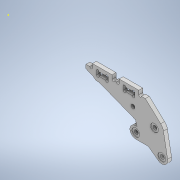
# Autodesk Inventor part: 後ろウィング固定フレーム
Saved by Autodesk Inventor 2020.2 (Build 242310000, 310)
## iProperties
Created: 2020-05-05
Part Number: 後ろウィング固定フレーム
Material: 一般
Document SubType Name: Modeling
Designer: mozar
Density: 1 g/cm^3
Appearance: 既定
Author: mozar
Autodesk Inventor part; units mm, degrees
ref_plane "YZ Plane" through (0, 0, 0) normal (1, 0, 0) x (0, 1, 0)
ref_plane "XZ Plane" through (0, 0, 0) normal (0, 1, 0) x (-1, 0, 0)
ref_plane "XY Plane" through (0, 0, 0) normal (0, 0, 1) x (1, 0, 0)
sketch "スケッチ2" plane through (0, 0, 0) normal (0, 0, 1) x (1, 0, 0)
  line L0 (-101.5, 47.999998) -> (108.5, 47.999998)
  circle A0 centre (111.885049, -19.000002) radius 4
  circle A1 centre (171.880735, -19.719469) radius 4
  circle A2 centre (111.885049, -19.000002) radius 7
  circle A3 centre (171.880735, -19.719469) radius 7
  line L1 (171.880735, -19.719469) -> (111.885049, -19.000002) construction
  line L2 (171.964673, -12.719973) -> (111.968987, -12.000505)
  line L3 (111.801111, -25.999499) -> (171.796797, -26.718966)
  arc A4 (171.796797, -26.718966) -> (171.964673, -12.719973) centre (171.880735, -19.719469) ccw
  arc A5 (111.968987, -12.000505) -> (111.801111, -25.999499) centre (111.885049, -19.000002) ccw
  line L4 (173.79611, -12.986614) -> (250.19065, -34.719469)
  circle A6 centre (241.981901, -63.574563) radius 30
  line L5 (268.180017, -78.191633) -> (221.951227, -41.241357)
  line L6 (221.951227, -41.241357) -> (169.96536, -26.452325)
  line L7 (271.981901, -113.136134) -> (271.981901, -54.819928)
  line L8 (111.885049, -19.000002) -> (111.885049, 40.999998) construction
  line L9 (118.885049, -19.000002) -> (118.885049, 40.999998)
  line L10 (104.885049, 40.999998) -> (104.885049, -19.000002)
  arc A7 (104.885049, -19.000002) -> (118.885049, -19.000002) centre (111.885049, -19.000002) ccw
  arc A8 (118.885049, 40.999998) -> (104.885049, 40.999998) centre (111.885049, 40.999998) ccw
  circle A9 centre (29.431847, 47.237971) radius 30
  line L11 (113.319325, 34.148513) -> (35.578743, 17.874462)
  line L12 (-0.558473, 47.999998) -> (57.548936, 36.777123)
  line L13 (57.548936, 36.777123) -> (110.450773, 47.851484)
  circle A10 centre (113.5, -20.000002) radius 68
  line L14 (321.963533, -82.955067) -> (60.270532, 100.284345)
  line L15 (259.189194, -39.000002) -> (111.885049, -19.000002)
  arc A11 (93.592427, -27.104845) -> (135.370976, -5.924402) centre (95.060351, 21.794105) ccw
  arc A12 (135.370976, -5.924402) -> (135.847591, -3.671647) centre (132.898992, -4.224609) ccw
  arc A13 (135.847591, -3.671647) -> (83.183341, 18.55647) centre (102.157897, -9.989602) ccw
  line L16 (111.885049, -19.000002) -> (112.689188, 40.994609) construction
  line L17 (118.88442, -19.093818) -> (119.688559, 40.900793)
  line L18 (105.689816, 41.088425) -> (104.885678, -18.906186)
  arc A14 (104.885678, -18.906186) -> (118.88442, -19.093818) centre (111.885049, -19.000002) ccw
  arc A15 (119.688559, 40.900793) -> (105.689816, 41.088425) centre (112.689188, 40.994609) ccw
  line L19 (164.994898, 47.999998) -> (164.994898, 25.999998)
  line L20 (164.994898, 25.999998) -> (327.494898, -102.000002)
  circle A16 centre (116.292557, -40.000002) radius 68
  circle A17 centre (-98.885049, -0.000002) radius 67.5
  line L21 (321.363327, -8.500986) -> (-152.668056, 78.49822)
  line L22 (104.889695, -3) -> (104.889695, 0)
  line L23 (104.889695, -3) -> (72.06562, -3)
  line L24 (72.06562, 0) -> (104.889695, 0)
  circle A18 centre (83.376901, -17.5) radius 13.85
  point P0 (0, 0)
  point P1 (141.882892, -19.359736)
  point P2 (111.885049, 10.999998)
  point P3 (105.885049, -0.000002)
  point P4 (105.885049, -0.000002)
  point P5 (23.732778, -42.728965)
  point P6 (112.287118, 10.997304)
  dimension "d31" = 8
  dimension "d32" = 8
  dimension "d33" = 3
  dimension "d34" = 3
  dimension "d35" = 60
  dimension "d36" = 14
  dimension "d37" = 14
  dimension "d38" = 60
  dimension "d39" = 14
  dimension "d40" = 60
  dimension "d41" = 14
  dimension "d42" = 6
  dimension "d43" = 35
  dimension "d44" = 13.271
  dimension "d45" = 14
  dimension "d46" = 20
  dimension "d47" = 15
  dimension "d48" = 22
  dimension "d49" = 150
  dimension "d50" = 162.5
  dimension "d51" = 0
  dimension "d52" = 136
  dimension "d53" = 136
  dimension "d54" = 135
  dimension "d55" = 38.2272
  dimension "d56" = 18
  constraints: 56 end point, 28 point on circle, 25 tangent, 18 centre point, 4 equal length, 3 coincident, 3 midpoint, 3 parallel, 3 vertical, 2 point on line, 1 concentric, 1 horizontal, 14 other
  measures "d31" diameter of A0
  measures "d32" diameter of A1
  measures "d33" radial gap between concentric circles of A0 A2
  measures "d35" distance of L1.start L1.end
  measures "d36" diameter of A5
  measures "d37" distance from line of L4 L5.end
  measures "d38" diameter of A6
  measures "d39" diameter of A8
  measures "d40" diameter of A9
  measures "d41" distance from line of L11 L12.end
  measures "d42" horizontal distance of L1.end point (105.885, 0)
  measures "d43" angle of L14 L0
  measures "d45" diameter of A15
  measures "d46" vertical distance of L15.start L1.end
  measures "d47" vertical distance of L1.start L4.end
  measures "d48" distance of L19.start L19.end
  measures "d49" vertical distance of L19.start L20.end
  measures "d50" distance from line of L19 L20.end
  measures "d51" distance from line of L19.start L0
  measures "d52" diameter of A10
  measures "d53" diameter of A16
  measures "d54" diameter of A17
  measures "d55" angle of L0 L20
  measures "d56" distance from line of L5.start L20
sketch "スケッチ1" plane through (0, 0, 0) normal (0, 0, 1) x (1, 0, 0)
  line L0 (-101.5, 47.999998) -> (108.5, 47.999998)
  circle A0 centre (111.885049, -19.000002) radius 4
  circle A1 centre (171.880735, -19.719469) radius 4
  circle A2 centre (111.885049, -19.000002) radius 7
  circle A3 centre (171.880735, -19.719469) radius 7
  line L1 (171.880735, -19.719469) -> (111.885049, -19.000002) construction
  line L2 (171.964673, -12.719973) -> (111.968987, -12.000505)
  line L3 (111.801111, -25.999499) -> (171.796797, -26.718966)
  arc A4 (171.796797, -26.718966) -> (171.964673, -12.719973) centre (171.880735, -19.719469) ccw
  arc A5 (111.968987, -12.000505) -> (111.801111, -25.999499) centre (111.885049, -19.000002) ccw
  line L4 (173.79611, -12.986614) -> (250.19065, -34.719469)
  circle A6 centre (241.981901, -63.574563) radius 30
  line L5 (268.180017, -78.191633) -> (221.951227, -41.241357)
  line L6 (221.951227, -41.241357) -> (169.96536, -26.452325)
  line L7 (271.981901, -113.136134) -> (271.981901, -54.819928)
  line L8 (111.885049, -19.000002) -> (111.885049, 40.999998) construction
  line L9 (118.885049, -19.000002) -> (118.885049, 40.999998)
  line L10 (104.885049, 40.999998) -> (104.885049, -19.000002)
  arc A7 (104.885049, -19.000002) -> (118.885049, -19.000002) centre (111.885049, -19.000002) ccw
  arc A8 (118.885049, 40.999998) -> (104.885049, 40.999998) centre (111.885049, 40.999998) ccw
  circle A9 centre (29.431847, 47.237971) radius 30
  line L11 (113.319325, 34.148513) -> (35.578743, 17.874462)
  line L12 (-0.558473, 47.999998) -> (57.548936, 36.777123)
  line L13 (57.548936, 36.777123) -> (110.450773, 47.851484)
  circle A10 centre (113.5, -20.000002) radius 68
  line L14 (321.963533, -82.955067) -> (60.270532, 100.284345)
  line L15 (259.189194, -39.000002) -> (111.885049, -19.000002)
  arc A11 (93.592427, -27.104845) -> (135.370976, -5.924402) centre (95.060351, 21.794105) ccw
  arc A12 (135.370976, -5.924402) -> (135.847591, -3.671647) centre (132.898992, -4.224609) ccw
  arc A13 (135.847591, -3.671647) -> (83.183341, 18.55647) centre (102.157897, -9.989602) ccw
  line L16 (111.885049, -19.000002) -> (112.689188, 40.994609) construction
  line L17 (118.88442, -19.093818) -> (119.688559, 40.900793)
  line L18 (105.689816, 41.088425) -> (104.885678, -18.906186)
  arc A14 (104.885678, -18.906186) -> (118.88442, -19.093818) centre (111.885049, -19.000002) ccw
  arc A15 (119.688559, 40.900793) -> (105.689816, 41.088425) centre (112.689188, 40.994609) ccw
  line L19 (164.994898, 47.999998) -> (164.994898, 25.999998)
  line L20 (164.994898, 25.999998) -> (327.494898, -102.000002)
  circle A16 centre (116.292557, -40.000002) radius 68
  circle A17 centre (-98.885049, -0.000002) radius 67.5
  line L21 (321.363327, -8.500986) -> (-152.668056, 78.49822)
  line L22 (104.889695, -3) -> (104.889695, 0)
  line L23 (72.06562, 0) -> (104.889695, 0)
  circle A18 centre (83.376901, -17.5) radius 13.85
  line L24 (104.889695, -3) -> (116.636882, -13.859955)
  line L25 (109.334849, -25.518934) -> (59.439695, -6)
  line L26 (94.885049, -3) -> (89.885049, -3)
  line L27 (87.885049, -3) -> (87.885049, -6)
  line L28 (89.885049, -6) -> (94.885049, -6)
  line L29 (96.885049, -6) -> (96.885049, -3)
  line L30 (74.439695, -3) -> (69.439695, -3)
  line L31 (67.439695, -3) -> (67.439695, -6)
  line L32 (69.439695, -6) -> (74.439695, -6)
  line L33 (76.439695, -6) -> (76.439695, -3)
  line L34 (59.439695, -3) -> (59.439695, -6)
  arc A19 (67.439695, -6) -> (69.439695, -6) centre (68.439695, -6) ccw
  arc A20 (74.439695, -6) -> (76.439695, -6) centre (75.439695, -6) ccw
  arc A21 (76.439695, -3) -> (74.439695, -3) centre (75.439695, -3) ccw
  arc A22 (69.439695, -3) -> (67.439695, -3) centre (68.439695, -3) ccw
  arc A23 (87.885049, -6) -> (89.885049, -6) centre (88.885049, -6) ccw
  arc A24 (94.885049, -6) -> (96.885049, -6) centre (95.885049, -6) ccw
  arc A25 (96.885049, -3) -> (94.885049, -3) centre (95.885049, -3) ccw
  arc A26 (89.885049, -3) -> (87.885049, -3) centre (88.885049, -3) ccw
  line L35 (104.889695, -3) -> (96.885049, -3)
  line L36 (94.885049, -3) -> (89.885049, -3)
  line L37 (87.885049, -3) -> (76.439695, -3)
  line L38 (74.439695, -3) -> (69.439695, -3)
  line L39 (67.439695, -3) -> (59.439695, -3)
  line L40 (84.885049, -3) -> (84.885049, -6)
  arc A27 (84.885049, -6) -> (91.5308, -9) centre (88.885049, -6) ccw
  line L41 (91.5308, -9) -> (93.239298, -9)
  arc A28 (93.239298, -9) -> (99.885049, -6) centre (95.885049, -6) ccw
  line L42 (99.885049, -6) -> (99.885049, -3)
  line L43 (79.439695, -3) -> (79.439695, -6)
  arc A29 (72.793944, -9) -> (79.439695, -6) centre (75.439695, -6) ccw
  line L44 (72.793944, -9) -> (71.085447, -9)
  arc A30 (64.439695, -6) -> (71.085447, -9) centre (68.439695, -6) ccw
  line L45 (64.439695, -6) -> (64.439695, -3)
  line L46 (84.885049, -3) -> (84.885049, 0)
  line L47 (84.885049, 0) -> (99.885049, 0)
  line L48 (99.885049, 0) -> (99.885049, -3)
  line L49 (87.885049, -3) -> (84.885049, -3)
  line L50 (99.885049, -3) -> (96.885049, -3)
  line L51 (94.885049, -3) -> (89.885049, -3)
  line L52 (64.439695, -3) -> (64.439695, 0)
  line L53 (64.439695, 0) -> (79.439695, 0)
  line L54 (79.439695, 0) -> (79.439695, -3)
  line L55 (79.439695, -3) -> (76.439695, -3)
  line L56 (74.439695, -3) -> (69.439695, -3)
  line L57 (67.439695, -3) -> (64.439695, -3)
  circle A31 centre (63.439695, -3) radius 1
  circle A32 centre (83.885049, -3) radius 1
  circle A33 centre (80.439695, -3) radius 1
  circle A34 centre (100.885049, -3) radius 1
  point P0 (0, 0)
  point P1 (141.882892, -19.359736)
  point P2 (111.885049, 10.999998)
  point P3 (105.885049, -0.000002)
  point P4 (105.885049, -0.000002)
  point P5 (23.732778, -42.728965)
  point P6 (112.287118, 10.997304)
  point P7 (104.889695, -1.5)
  point P8 (101.885049, -3)
  point P9 (82.885049, -3)
  point P10 (81.439695, -3)
  point P11 (62.439695, -3)
  point P12 (65.111495, -8.218802)
  point P13 (69.378847, -9.888186)
  point P14 (108.577071, -25.222492)
  point P15 (108.642416, -25.203657)
  dimension "d0" = 8
  dimension "d1" = 8
  dimension "d2" = 3
  dimension "d3" = 3
  dimension "d4" = 60
  dimension "d5" = 14
  dimension "d6" = 14
  dimension "d7" = 60
  dimension "d8" = 14
  dimension "d9" = 60
  dimension "d10" = 14
  dimension "d11" = 6
  dimension "d12" = 35
  dimension "d13" = 13.271
  dimension "d14" = 14
  dimension "d15" = 20
  dimension "d16" = 15
  dimension "d17" = 22
  dimension "d18" = 150
  dimension "d19" = 162.5
  dimension "d20" = 0
  dimension "d21" = 136
  dimension "d22" = 136
  dimension "d23" = 135
  dimension "d24" = 38.2272
  dimension "d25" = 18
  dimension "d26" = 9
  dimension "d27" = 3
  dimension "d28" = 9
  dimension "d29" = 3
  dimension "d30" = 8
  dimension "d57" = 45.45
  dimension "d58" = 3
  dimension "d60" = 2
  dimension "d61" = 2
  dimension "d62" = 2
  dimension "d63" = 2
  dimension "d64" = 2
  dimension "d65" = 2
  dimension "d66" = 2
  dimension "d67" = 2
  dimension "d68" = 3
  dimension "d69" = 3
  dimension "d73" = 8
  dimension "d74" = 2
  dimension "d75" = 2
  dimension "d76" = 2
  dimension "d77" = 2
  constraints: 122 end point, 53 point on circle, 37 tangent, 33 centre point, 17 parallel, 17 point on line, 15 horizontal, 8 perpendicular, 5 midpoint, 5 vertical, 4 equal length, 3 coincident, 30 other
  measures "d0" diameter of A0
  measures "d1" diameter of A1
  measures "d4" distance of L1.start L1.end
  measures "d5" diameter of A5
  measures "d6" distance from line of L4 L5.end
  measures "d7" diameter of A6
  measures "d8" diameter of A8
  measures "d9" diameter of A9
  measures "d10" distance from line of L11 L12.end
  measures "d11" horizontal distance of L1.end point (105.885, 0)
  measures "d12" angle of L14 L0
  measures "d14" diameter of A15
  measures "d15" vertical distance of L15.start L1.end
  measures "d16" vertical distance of L1.start L4.end
  measures "d17" distance of L19.start L19.end
  measures "d18" vertical distance of L19.start L20.end
  measures "d19" distance from line of L19 L20.end
  measures "d20" distance from line of L19.start L0
  measures "d21" diameter of A10
  measures "d22" diameter of A16
  measures "d23" diameter of A17
  measures "d24" angle of L0 L20
  measures "d25" distance from line of L5.start L20
  measures "d26" distance of L29.start L27.end
  measures "d27" distance of L27.end L27.start
  measures "d28" distance of L33.start L31.end
  measures "d29" distance of L31.end L31.start
  measures "d30" distance between parallel lines of L29 L10
  measures "d57" distance from line of L34.start L22
  measures "d58" distance of L34.start L25.end
  measures "d60" diameter of A19
  measures "d61" diameter of A20
  measures "d62" diameter of A21
  measures "d63" diameter of A22
  measures "d64" diameter of A23
  measures "d65" diameter of A24
  measures "d66" diameter of A25
  measures "d67" diameter of A26
  measures "d68" distance between parallel lines of L27 L40
  measures "d69" distance between parallel lines of L33 L43
  measures "d73" distance between parallel lines of L34 L31
  measures "d74" diameter of A31
  measures "d75" diameter of A32
  measures "d76" diameter of A33
  measures "d77" diameter of A34
extrude "押し出し1" add sketch "スケッチ1" against normal blind 3 contours A2 A11 | L35 L24 L18 L10 | L10 A2 A11 L25 A18 A28 L42 A34 L35 | L48 L35 A25 L26 A26 L37 L46 L23 | L24 L2 A2 L18 | A11 A2 | L42 A28 A18 L28 A24 L29 L35 | L24 A2 L2 | L54 L37 A21 L30 A22 L39 L52 L53 L23 | L37 L27 A18 L40 | L40 A18 A32 | L25 A18 L44 A29 L43 A33 A32 L40 A27 L41 A28 | L43 A18 L33 L37 | A33 A18 L43 | A32 A18 A33 L37 | A18 L27 A23 L28 A28 L41 A27 L40 | L25 A30 L44 A18 | L43 A29 L44 A18 A20 L33 | L44 A30 L25 L45 L39 L31 A19 L32 A20 A18 | A30 L25 | L45 A30 L25 L34 L39 A31 | A0
hole "穴1" at (111.885049, -19.000002, 0) direction (0, 0, -1) diameter 3 depth 12 tip angle 118
sketch "スケッチ3" plane through (0, 0, 0) normal (0, 0, 1) x (1, 0, 0)
  circle A0 centre (111.885049, -19.000002) radius 1.5
  line L0 (89.885049, -6) -> (94.885049, -6)
  arc A1 (94.885049, -6) -> (96.885049, -6) centre (95.885049, -6) ccw
  line L1 (96.885049, -6) -> (96.885049, -3)
  arc A2 (96.885049, -3) -> (94.885049, -3) centre (95.885049, -3) ccw
  line L2 (94.885049, -3) -> (89.885049, -3)
  arc A3 (89.885049, -3) -> (87.885049, -3) centre (88.885049, -3) ccw
  line L3 (87.885049, -3) -> (87.885049, -6)
  arc A4 (87.885049, -6) -> (89.885049, -6) centre (88.885049, -6) ccw
  arc A5 (76.439695, -3) -> (74.439695, -3) centre (75.439695, -3) ccw
  line L4 (74.439695, -3) -> (69.439695, -3)
  arc A6 (69.439695, -3) -> (67.439695, -3) centre (68.439695, -3) ccw
  line L5 (67.439695, -3) -> (67.439695, -6)
  arc A7 (67.439695, -6) -> (69.439695, -6) centre (68.439695, -6) ccw
  line L6 (69.439695, -6) -> (74.439695, -6)
  arc A8 (74.439695, -6) -> (76.439695, -6) centre (75.439695, -6) ccw
  line L7 (76.439695, -6) -> (76.439695, -3)
  line L8 (64.439695, -3) -> (64.439695, 0)
  line L9 (64.439695, 0) -> (79.439695, 0)
  line L10 (79.439695, 0) -> (79.439695, -3)
  arc A9 (79.439695, -3) -> (81.439695, -3) centre (80.439695, -3) ccw
  line L11 (81.439695, -3) -> (82.885049, -3)
  arc A10 (82.885049, -3) -> (84.885049, -3) centre (83.885049, -3) ccw
  line L12 (84.885049, -3) -> (84.885049, 0)
  line L13 (84.885049, 0) -> (99.885049, 0)
  line L14 (99.885049, 0) -> (99.885049, -3)
  arc A11 (99.885049, -3) -> (101.885049, -3) centre (100.885049, -3) ccw
  line L15 (101.885049, -3) -> (104.889695, -3)
  line L16 (104.889695, -3) -> (116.636882, -13.859955)
  arc A12 (108.642416, -25.203657) -> (116.636882, -13.859955) centre (111.885049, -19.000002) ccw
  arc A13 (108.577071, -25.222492) -> (108.642416, -25.203657) centre (95.060351, 21.794105) ccw
  line L17 (108.577071, -25.222492) -> (69.378847, -9.888186)
  arc A14 (65.111495, -8.218802) -> (69.378847, -9.888186) centre (68.439695, -6) ccw
  line L18 (65.111495, -8.218802) -> (59.439695, -6)
  line L19 (59.439695, -6) -> (59.439695, -3)
  line L20 (59.439695, -3) -> (62.439695, -3)
  arc A15 (62.439695, -3) -> (64.439695, -3) centre (63.439695, -3) ccw
  circle A16 centre (111.885049, -19.000002) radius 9
  circle A17 centre (111.885049, -19.000002) radius 9.5
  line L21 (111.801111, -25.999499) -> (171.796797, -26.718966)
  circle A18 centre (111.885049, -19.000002) radius 14.5
  line L22 (111.741155, -30.999139) -> (171.736842, -31.718607)
  line L23 (93.239298, -9) -> (91.5308, -9)
  arc A19 (84.885049, -6) -> (91.5308, -9) centre (88.885049, -6) ccw
  line L24 (84.885049, -6) -> (84.885049, -3)
  arc A20 (91.5308, 0) -> (84.885049, -3) centre (88.885049, -3) ccw
  line L25 (91.5308, 0) -> (93.239298, 0)
  arc A21 (99.885049, -3) -> (93.239298, 0) centre (95.885049, -3) ccw
  line L26 (99.885049, -3) -> (99.885049, -6)
  arc A22 (93.239298, -9) -> (99.885049, -6) centre (95.885049, -6) ccw
  line L27 (72.793944, -9) -> (71.085447, -9)
  arc A23 (64.439695, -6) -> (71.085447, -9) centre (68.439695, -6) ccw
  line L28 (64.439695, -6) -> (64.439695, -3)
  arc A24 (71.085447, 0) -> (64.439695, -3) centre (68.439695, -3) ccw
  line L29 (71.085447, 0) -> (72.793944, 0)
  arc A25 (79.439695, -3) -> (72.793944, 0) centre (75.439695, -3) ccw
  line L30 (79.439695, -3) -> (79.439695, -6)
  arc A26 (72.793944, -9) -> (79.439695, -6) centre (75.439695, -6) ccw
  line L31 (69.232457, -6.609532) -> (108.707488, -22.052125)
  arc A27 (108.707488, -22.052125) -> (109.14454, -21.913696) centre (95.060351, 21.794105) ccw
  arc A28 (109.14454, -21.913696) -> (114.600382, -16.062832) centre (111.885049, -19.000002) ccw
  line L32 (114.600382, -16.062832) -> (103.715441, -6)
  line L33 (103.715441, -6) -> (103.5308, -6)
  arc A29 (96.885049, -3) -> (103.5308, -6) centre (100.885049, -3) ccw
  line L34 (96.885049, -3) -> (87.885049, -3)
  arc A30 (82.162372, -6.610039) -> (87.885049, -3) centre (83.885049, -3) ccw
  arc A31 (76.439695, -3) -> (82.162372, -6.610039) centre (80.439695, -3) ccw
  line L35 (76.439695, -3) -> (67.439695, -3)
  arc A32 (66.522117, -5.54925) -> (67.439695, -3) centre (63.439695, -3) ccw
  line L36 (66.522117, -5.54925) -> (67.443772, -5.9098)
  arc A33 (67.443772, -5.9098) -> (69.232457, -6.609532) centre (68.439695, -6) ccw
  circle A34 centre (111.885049, -19.000002) radius 1.5
  line L37 (111.885049, -19.000002) -> (111.885049, 12.517364) construction
  line L38 (118.885049, -19.000002) -> (118.885049, 12.517364)
  line L39 (104.885049, 12.517364) -> (104.885049, -19.000002)
  arc A35 (104.885049, -19.000002) -> (118.885049, -19.000002) centre (111.885049, -19.000002) ccw
  arc A36 (118.885049, 12.517364) -> (104.885049, 12.517364) centre (111.885049, 12.517364) ccw
  circle A37 centre (95.450697, -12.986511) radius 3
  circle A38 centre (117.517728, -35.568735) radius 4.5
  circle A39 centre (71.939695, -13.745967) radius 4.5
  line L40 (114.848974, -39.191959) -> (103.285731, -30.674835)
  line L41 (106.485085, -32.456985) -> (70.263844, -17.922272)
  line L42 (121.941475, -34.743835) -> (118.766434, -17.716824)
  arc A40 (108.642416, -25.203657) -> (116.636882, -13.859955) centre (111.885049, -19.000002) ccw
  circle A41 centre (117.517728, -35.568735) radius 3
  circle A42 centre (97.594486, -29.100982) radius 3
  circle A43 centre (97.594486, -29.100982) radius 4.5
  circle A44 centre (83.376901, -17.5) radius 13.85
  line L43 (111.987254, -33.499642) -> (97.626204, -33.60087)
  point P0 (0, 0)
  point P1 (111.885049, -3.241319)
  point P2 (69.528251, -9.946633)
  point P3 (118.885049, -18.352931)
  point P4 (118.766434, -17.716824)
  point P5 (121.094196, -30.200074)
  point P6 (104.771972, -31.769554)
  point P7 (97.50911, -20.892717)
  point P8 (107.312526, -5.239841)
  point P9 (104.885049, -6.301577)
  point P10 (104.885049, -3)
  point P11 (98.554323, -24.704539)
  point P12 (107.166949, -33.533619)
  dimension "d104" = 9
  dimension "d128" = 9
  dimension "d91" = 18
  dimension "d92" = 0.5
  dimension "d93" = 5
  dimension "d94" = 5
  dimension "d96" = 3
  dimension "d97" = 3
  dimension "d98" = 3
  dimension "d99" = 14
  dimension "d102" = 6
  dimension "d103" = 9
  dimension "d126" = 6
  dimension "d127" = 6
  constraints: 46 end point, 40 point on circle, 24 centre point, 15 tangent, 3 coincident, 2 parallel, 1 midpoint, 1 vertical, 37 other
  measures "d91" diameter of A16
  measures "d92" radial gap between concentric circles of A16 A17
  measures "d93" radial gap between concentric circles of A17 A18
  measures "d94" distance between parallel lines of L21 L22
  measures "d96" distance between parallel lines of L0 L23
  measures "d97" distance between parallel lines of L6 L27
  measures "d98" distance between parallel lines of L17 L31
  measures "d99" diameter of A36
  measures "d102" diameter of A37
  measures "d103" diameter of A38
  measures "d126" diameter of A41
  measures "d127" diameter of A42
sketch "スケッチ3 outline for 押し出し2" plane through (0, 0, 0) normal (0, 0, 1) x (1, 0, 0)
  line L0 (116.636882, -13.859955) -> (107.312526, -5.239841)
  arc A0 (107.312526, -5.239841) -> (98.554323, -24.704539) centre (111.885049, -19.000002) ccw
  arc A1 (98.554323, -24.704539) -> (97.626204, -33.60087) centre (97.594486, -29.100982) ccw
  line L1 (97.626204, -33.60087) -> (107.166949, -33.533619)
  line L2 (107.166949, -33.533619) -> (114.848974, -39.191959)
  arc A2 (114.848974, -39.191959) -> (121.941475, -34.743835) centre (117.517728, -35.568735) ccw
  line L3 (121.941475, -34.743835) -> (118.766434, -17.716824)
  arc A3 (118.766434, -17.716824) -> (116.636882, -13.859955) centre (111.885049, -19.000002) ccw
  circle A4 centre (111.885049, -19.000002) radius 1.5
extrude "押し出し2" add sketch "スケッチ3 outline for 押し出し2" against normal blind 3
hole "穴2" at (71.939695, -13.745967, 0) at (95.450697, -12.986511, 0) at (117.517728, -35.568735, 0) at (97.594486, -29.100982, 0) direction (0, 0, -1) diameter 3 depth 12 tip angle 118
sketch "スケッチ4" plane through (0, 0, 0) normal (0, 0, 1) x (1, 0, 0)
  circle A0 centre (111.885049, -19.000002) radius 1.5
  line L0 (89.885049, -6) -> (94.885049, -6)
  arc A1 (94.885049, -6) -> (96.885049, -6) centre (95.885049, -6) ccw
  line L1 (96.885049, -6) -> (96.885049, -3)
  arc A2 (96.885049, -3) -> (94.885049, -3) centre (95.885049, -3) ccw
  line L2 (94.885049, -3) -> (89.885049, -3)
  arc A3 (89.885049, -3) -> (87.885049, -3) centre (88.885049, -3) ccw
  line L3 (87.885049, -3) -> (87.885049, -6)
  arc A4 (87.885049, -6) -> (89.885049, -6) centre (88.885049, -6) ccw
  arc A5 (76.439695, -3) -> (74.439695, -3) centre (75.439695, -3) ccw
  line L4 (74.439695, -3) -> (69.439695, -3)
  arc A6 (69.439695, -3) -> (67.439695, -3) centre (68.439695, -3) ccw
  line L5 (67.439695, -3) -> (67.439695, -6)
  arc A7 (67.439695, -6) -> (69.439695, -6) centre (68.439695, -6) ccw
  line L6 (69.439695, -6) -> (74.439695, -6)
  arc A8 (74.439695, -6) -> (76.439695, -6) centre (75.439695, -6) ccw
  line L7 (76.439695, -6) -> (76.439695, -3)
  line L8 (64.439695, -3) -> (64.439695, 0)
  line L9 (64.439695, 0) -> (79.439695, 0)
  line L10 (79.439695, 0) -> (79.439695, -3)
  arc A9 (79.439695, -3) -> (81.439695, -3) centre (80.439695, -3) ccw
  line L11 (81.439695, -3) -> (82.885049, -3)
  arc A10 (82.885049, -3) -> (84.885049, -3) centre (83.885049, -3) ccw
  line L12 (84.885049, -3) -> (84.885049, 0)
  line L13 (84.885049, 0) -> (99.885049, 0)
  line L14 (99.885049, 0) -> (99.885049, -3)
  arc A11 (99.885049, -3) -> (101.885049, -3) centre (100.885049, -3) ccw
  line L15 (101.885049, -3) -> (104.889695, -3)
  line L16 (104.889695, -3) -> (116.636882, -13.859955)
  arc A12 (108.642416, -25.203657) -> (116.636882, -13.859955) centre (111.885049, -19.000002) ccw
  arc A13 (108.577071, -25.222492) -> (108.642416, -25.203657) centre (95.060351, 21.794105) ccw
  line L17 (108.577071, -25.222492) -> (69.378847, -9.888186)
  arc A14 (65.111495, -8.218802) -> (69.378847, -9.888186) centre (68.439695, -6) ccw
  line L18 (65.111495, -8.218802) -> (59.439695, -6)
  line L19 (59.439695, -6) -> (59.439695, -3)
  line L20 (59.439695, -3) -> (62.439695, -3)
  arc A15 (62.439695, -3) -> (64.439695, -3) centre (63.439695, -3) ccw
  circle A16 centre (111.885049, -19.000002) radius 9
  circle A17 centre (111.885049, -19.000002) radius 9.5
  line L21 (111.801111, -25.999499) -> (171.796797, -26.718966)
  circle A18 centre (111.885049, -19.000002) radius 14.5
  line L22 (111.741155, -30.999139) -> (171.736842, -31.718607)
  line L23 (93.239298, -9) -> (91.5308, -9)
  arc A19 (84.885049, -6) -> (91.5308, -9) centre (88.885049, -6) ccw
  line L24 (84.885049, -6) -> (84.885049, -3)
  arc A20 (91.5308, 0) -> (84.885049, -3) centre (88.885049, -3) ccw
  line L25 (91.5308, 0) -> (93.239298, 0)
  arc A21 (99.885049, -3) -> (93.239298, 0) centre (95.885049, -3) ccw
  line L26 (99.885049, -3) -> (99.885049, -6)
  arc A22 (93.239298, -9) -> (99.885049, -6) centre (95.885049, -6) ccw
  line L27 (72.793944, -9) -> (71.085447, -9)
  arc A23 (64.439695, -6) -> (71.085447, -9) centre (68.439695, -6) ccw
  line L28 (64.439695, -6) -> (64.439695, -3)
  arc A24 (71.085447, 0) -> (64.439695, -3) centre (68.439695, -3) ccw
  line L29 (71.085447, 0) -> (72.793944, 0)
  arc A25 (79.439695, -3) -> (72.793944, 0) centre (75.439695, -3) ccw
  line L30 (79.439695, -3) -> (79.439695, -6)
  arc A26 (72.793944, -9) -> (79.439695, -6) centre (75.439695, -6) ccw
  line L31 (69.232457, -6.609532) -> (108.707488, -22.052125)
  arc A27 (108.707488, -22.052125) -> (109.14454, -21.913696) centre (95.060351, 21.794105) ccw
  arc A28 (109.14454, -21.913696) -> (114.600382, -16.062832) centre (111.885049, -19.000002) ccw
  line L32 (114.600382, -16.062832) -> (103.715441, -6)
  line L33 (103.715441, -6) -> (103.5308, -6)
  arc A29 (96.885049, -3) -> (103.5308, -6) centre (100.885049, -3) ccw
  line L34 (96.885049, -3) -> (87.885049, -3)
  arc A30 (82.162372, -6.610039) -> (87.885049, -3) centre (83.885049, -3) ccw
  arc A31 (76.439695, -3) -> (82.162372, -6.610039) centre (80.439695, -3) ccw
  line L35 (76.439695, -3) -> (67.439695, -3)
  arc A32 (66.522117, -5.54925) -> (67.439695, -3) centre (63.439695, -3) ccw
  line L36 (66.522117, -5.54925) -> (67.443772, -5.9098)
  arc A33 (67.443772, -5.9098) -> (69.232457, -6.609532) centre (68.439695, -6) ccw
  circle A34 centre (111.885049, -19.000002) radius 1.5
  line L37 (111.885049, -19.000002) -> (111.885049, 12.517364) construction
  line L38 (118.885049, -19.000002) -> (118.885049, 12.517364)
  line L39 (104.885049, 12.517364) -> (104.885049, -19.000002)
  arc A35 (104.885049, -19.000002) -> (118.885049, -19.000002) centre (111.885049, -19.000002) ccw
  arc A36 (118.885049, 12.517364) -> (104.885049, 12.517364) centre (111.885049, 12.517364) ccw
  circle A37 centre (95.450697, -12.986511) radius 3
  circle A38 centre (121.10724, -35.611781) radius 4.5
  circle A39 centre (71.939695, -13.745967) radius 4.5
  line L40 (118.911469, -39.539705) -> (104.809788, -31.656648)
  line L41 (106.485085, -32.456985) -> (70.263844, -17.922272)
  line L42 (125.294797, -33.964248) -> (118.399027, -16.437173)
  arc A40 (108.642416, -25.203657) -> (116.636882, -13.859955) centre (111.885049, -19.000002) ccw
  point P0 (0, 0)
  point P1 (0, 0)
  point P2 (111.885049, -3.241319)
  point P3 (69.528251, -9.946633)
  point P4 (118.885049, -17.672502)
  point P5 (118.399027, -16.437173)
  point P6 (123.048154, -28.253924)
  point P7 (105.621764, -32.110555)
  point P8 (97.50911, -20.892717)
  point P9 (107.312526, -5.239841)
  point P10 (104.885049, -6.301577)
  point P11 (104.885049, -3)
  dimension "d124" = 9
  dimension "d114" = 18
  dimension "d115" = 0.5
  dimension "d116" = 5
  dimension "d117" = 5
  dimension "d118" = 3
  dimension "d119" = 3
  dimension "d120" = 3
  dimension "d121" = 14
  dimension "d122" = 6
  dimension "d123" = 9
  constraints: 88 end point, 71 point on circle, 40 centre point, 13 tangent, 2 parallel, 1 coincident, 1 midpoint, 1 vertical, 32 other
  measures "d114" diameter of A16
  measures "d115" radial gap between concentric circles of A16 A17
  measures "d116" radial gap between concentric circles of A17 A18
  measures "d117" distance between parallel lines of L21 L22
  measures "d118" distance between parallel lines of L0 L23
  measures "d119" distance between parallel lines of L6 L27
  measures "d120" distance between parallel lines of L17 L31
  measures "d121" diameter of A36
  measures "d122" diameter of A37
  measures "d123" diameter of A38
sketch "スケッチ5" plane through (0, 0, 0) normal (0, 0, 1) x (1, 0, 0)
  circle A0 centre (117.517728, -35.568735) radius 1.5
  circle A1 centre (95.450697, -12.986511) radius 1.5
  circle A2 centre (97.594486, -29.100982) radius 1.5
  circle A3 centre (111.885049, -19.000002) radius 1.5
  line L0 (116.636882, -13.859955) -> (104.889695, -3)
  line L1 (104.889695, -3) -> (101.885049, -3)
  arc A4 (99.885049, -3) -> (101.885049, -3) centre (100.885049, -3) ccw
  line L2 (99.885049, -3) -> (99.885049, 0)
  line L3 (99.885049, 0) -> (84.885049, 0)
  line L4 (84.885049, 0) -> (84.885049, -3)
  arc A5 (82.885049, -3) -> (84.885049, -3) centre (83.885049, -3) ccw
  line L5 (82.885049, -3) -> (81.439695, -3)
  arc A6 (79.439695, -3) -> (81.439695, -3) centre (80.439695, -3) ccw
  line L6 (79.439695, -3) -> (79.439695, 0)
  line L7 (79.439695, 0) -> (64.439695, 0)
  line L8 (64.439695, 0) -> (64.439695, -3)
  arc A7 (62.439695, -3) -> (64.439695, -3) centre (63.439695, -3) ccw
  line L9 (62.439695, -3) -> (59.439695, -3)
  line L10 (59.439695, -3) -> (59.439695, -6)
  line L11 (59.439695, -6) -> (65.111495, -8.218802)
  arc A8 (65.111495, -8.218802) -> (69.378847, -9.888186) centre (68.439695, -6) ccw
  line L12 (69.378847, -9.888186) -> (97.50911, -20.892717)
  arc A9 (97.50911, -20.892717) -> (98.554323, -24.704539) centre (111.885049, -19.000002) ccw
  arc A10 (98.554323, -24.704539) -> (97.626204, -33.60087) centre (97.594486, -29.100982) ccw
  line L13 (97.626204, -33.60087) -> (107.166949, -33.533619)
  line L14 (107.166949, -33.533619) -> (114.848974, -39.191959)
  arc A11 (114.848974, -39.191959) -> (121.941475, -34.743835) centre (117.517728, -35.568735) ccw
  line L15 (121.941475, -34.743835) -> (118.766434, -17.716824)
  arc A12 (118.766434, -17.716824) -> (116.636882, -13.859955) centre (111.885049, -19.000002) ccw
  line L16 (69.439695, -3) -> (74.439695, -3)
  arc A13 (76.439695, -3) -> (74.439695, -3) centre (75.439695, -3) ccw
  line L17 (76.439695, -3) -> (76.439695, -6)
  arc A14 (74.439695, -6) -> (76.439695, -6) centre (75.439695, -6) ccw
  line L18 (74.439695, -6) -> (69.439695, -6)
  arc A15 (67.439695, -6) -> (69.439695, -6) centre (68.439695, -6) ccw
  line L19 (67.439695, -6) -> (67.439695, -3)
  arc A16 (69.439695, -3) -> (67.439695, -3) centre (68.439695, -3) ccw
  arc A17 (94.885049, -6) -> (96.885049, -6) centre (95.885049, -6) ccw
  line L20 (94.885049, -6) -> (89.885049, -6)
  arc A18 (87.885049, -6) -> (89.885049, -6) centre (88.885049, -6) ccw
  line L21 (87.885049, -6) -> (87.885049, -3)
  arc A19 (89.885049, -3) -> (87.885049, -3) centre (88.885049, -3) ccw
  line L22 (89.885049, -3) -> (94.885049, -3)
  arc A20 (96.885049, -3) -> (94.885049, -3) centre (95.885049, -3) ccw
  line L23 (96.885049, -3) -> (96.885049, -6)
  circle A21 centre (117.517728, -35.568735) radius 1.5
  circle A22 centre (117.517728, -35.568735) radius 3
  circle A23 centre (97.594486, -29.100982) radius 1.5
  circle A24 centre (97.594486, -29.100982) radius 3
  circle A25 centre (111.885049, -19.000002) radius 1.5
  circle A26 centre (111.885049, -19.000002) radius 3
  point P0 (0, 0)
  dimension "d129" = 6
  dimension "d130" = 6
  dimension "d133" = 6
  constraints: 3 centre point, 3 coincident
  measures "d129" diameter of A22
  measures "d130" diameter of A24
  measures "d133" diameter of A26
extrude "押し出し3" cut sketch "スケッチ5" against normal blind 0.4 contours A0 | A2 | A22 | A24 | A26
sketch "スケッチ6" plane through (0, 0, 0) normal (0, 0, 1) x (1, 0, 0)
  point P0 (0, 0)
equation "\"d40\" = d38"
equation "\"d9\" = d7"
